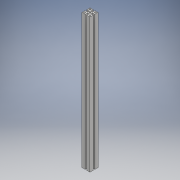
# Autodesk Inventor part: 3030500
Saved by Autodesk Inventor 2018 (Build 220112000, 112)
## iProperties
Created: 2020-09-14
Part Number: 3030500
Material: 일반
Document SubType Name: Sheet Metal
Designer: j3jjj
Density: 1 g/cm^3
Sheet Metal Rule: 기본값_mm
Appearance: 기본값
Author: j3jjj
Autodesk Inventor part; units mm, degrees
ref_plane "YZ Plane" through (0, 0, 0) normal (1, 0, 0) x (0, 1, 0)
ref_plane "XZ Plane" through (0, 0, 0) normal (0, 1, 0) x (-1, 0, 0)
ref_plane "XY Plane" through (0, 0, 0) normal (0, 0, 1) x (1, 0, 0)
sketch "스케치1" plane through (0, 0, 0) normal (0, 0, 1) x (1, 0, 0)
  line L0 (15, 15) -> (-15, 15)
  line L1 (-15, 15) -> (-15, -15)
  line L2 (-15, -15) -> (15, -15)
  line L3 (15, -15) -> (15, 15)
  circle A0 centre (0, 0) radius 2.5
  circle A1 centre (-10, 10) radius 3
  circle A2 centre (10, 10) radius 3
  circle A3 centre (10, -10) radius 3
  circle A4 centre (-10, -10) radius 3
  line L4 (3.15, 15) -> (-3.15, 15)
  line L5 (-3.15, 15) -> (-3.15, 5)
  line L6 (-3.15, 5) -> (3.15, 5)
  line L7 (3.15, 5) -> (3.15, 15)
  line L8 (-15, -3.15) -> (-5, -3.15)
  line L9 (-5, 3.15) -> (-15, 3.15)
  line L10 (-5, -3.15) -> (-5, 3.15)
  line L11 (-15, 3.15) -> (-15, -3.15)
  line L12 (3.15, -15) -> (3.15, -5)
  line L13 (-3.15, -5) -> (-3.15, -15)
  line L14 (3.15, -5) -> (-3.15, -5)
  line L15 (-3.15, -15) -> (3.15, -15)
  line L16 (15, 3.15) -> (5, 3.15)
  line L17 (5, -3.15) -> (15, -3.15)
  line L18 (5, 3.15) -> (5, -3.15)
  line L19 (15, -3.15) -> (15, 3.15)
  dimension "d0" = 30
  dimension "d1" = 15
  dimension "d2" = 30
  dimension "d3" = 15
  dimension "d4" = 20
  dimension "d5" = 10
  dimension "d6" = 20
  dimension "d7" = 10
  dimension "d8" = 20
  dimension "d9" = 20
  dimension "d10" = 10
  dimension "d11" = 10
  dimension "d12" = 6
  dimension "d13" = 6
  dimension "d14" = 6
  dimension "d15" = 6
  dimension "d16" = 5
  dimension "d17" = 0
  dimension "d18" = 6.3
  dimension "d19" = 3.15
  dimension "d20" = 10
  dimension "d23" = 360
  constraints: 40 end point, 5 centre point, 4 parallel, 2 horizontal, 2 perpendicular, 1 coincident, 33 other
  measures "d0" distance between parallel lines of L3 L1
  measures "d1" distance from line of point (0, 0) L1
  measures "d2" distance between parallel lines of L2 L0
  measures "d3" distance from line of point (0, 0) L0
  measures "d4" distance of A4.centre A1.centre
  measures "d5" horizontal distance of point (0, 0) A1.centre
  measures "d6" distance of A2.centre A1.centre
  measures "d7" horizontal distance of A2.centre point (0, 0)
  measures "d8" distance of A3.centre A2.centre
  measures "d9" distance of A3.centre A4.centre
  measures "d10" horizontal distance of point (0, 0) A4.centre
  measures "d11" horizontal distance of A2.centre point (0, 0)
  measures "d12" diameter of A2
  measures "d13" diameter of A3
  measures "d14" diameter of A4
  measures "d15" diameter of A1
  measures "d16" diameter of A0
  measures "d17" distance between parallel lines of L4 L0
  measures "d18" distance between parallel lines of L7 L5
  measures "d19" distance from line of point (0, 0) L5
  measures "d20" distance between parallel lines of L6 L4
extrude "돌출1" add sketch "스케치1" along normal blind 500 contours L3 L16 L18 L17 L2 L12 L14 L13 L1 L8 L10 L9 L0 L5 L6 L7
equation "\"TransitionRadius\" = BendRadius"
equation "\"BendRadius\" = 0.5"
